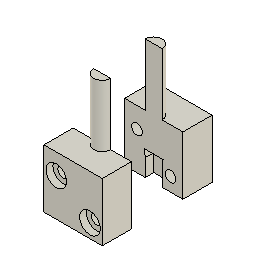
fl57sth76_gt2_adapter (Autodesk Fusion 360 design; units mm, degrees)
Autodesk Fusion 360 part; units mm, degrees
note: some values were not read from the file. Chosen so that the rebuilt part matches the saved one: which bodies a step acts on.
sketch "Sketch1" plane through (0, 0, 0) normal (0, 0, 1) x (1, 0, 0)
  line L0 (2.5, 2.5) -> (-2.5, 2.5)
  line L1 (-2.5, 2.5) -> (-2.5, -2.5)
  line L2 (-2.5, -2.5) -> (2.5, -2.5)
  line L3 (2.5, -2.5) -> (2.5, 2.5)
  line L4 (2.5, 2.5) -> (-2.5, -2.5) construction
  line L5 (-2.5, 2.5) -> (2.5, -2.5) construction
  dimension "d1" = 5
  dimension "d2" = 5
  constraint horizontal L0
  constraint perpendicular L0 L1
  constraint parallel L0 L2
  constraint parallel L1 L3
  constraint coincident L4 origin
  constraint coincident L5 origin
  measures "d1" distance of L1.end L2.end
  measures "d2" distance of L0.end L1.end
extrude "Extrude1" add sketch "Sketch1" along normal blind 5 makes body 1
ref_plane "WorkPlane1" through (0, 0, 7.15) normal (0, 0, 1) x (1, 0, 0)
sketch "Sketch2" plane through (0, 0, 7.15) normal (0, 0, 1) x (1, 0, 0)
  line L0 (2.675, 2.675) -> (-2.675, 2.675)
  line L1 (-2.675, 2.675) -> (-2.675, -2.675)
  line L2 (-2.675, -2.675) -> (2.675, -2.675)
  line L3 (2.675, -2.675) -> (2.675, 2.675)
  line L4 (2.675, 2.675) -> (-2.675, -2.675) construction
  line L5 (-2.675, 2.675) -> (2.675, -2.675) construction
  dimension "d7" = 5.35
  dimension "d8" = 5.35
  constraint horizontal L0
  constraint perpendicular L0 L1
  constraint parallel L0 L2
  constraint parallel L1 L3
  constraint coincident L4 origin
  constraint coincident L5 origin
  measures "d7" distance of L1.end L2.end
  measures "d8" distance of L0.end L1.end
loft "Loft1" add profiles "Sketch2" section 1 face at (-0.8333, 0.8333, 5) section 2 on bodies 1 bodies 1
sketch "Sketch3" plane through (0, 0, 0) normal (0, 0, 1) x (1, 0, 0)
  line L0 (8.5, 8.5) -> (-8.5, 8.5)
  line L1 (-8.5, 8.5) -> (-8.5, -8.5)
  line L2 (-8.5, -8.5) -> (8.5, -8.5)
  line L3 (8.5, -8.5) -> (8.5, 8.5)
  line L4 (8.5, 8.5) -> (-8.5, -8.5) construction
  line L5 (-8.5, 8.5) -> (8.5, -8.5) construction
  dimension "d9" = 17
  dimension "d10" = 17
  constraint horizontal L0
  constraint perpendicular L0 L1
  constraint parallel L0 L2
  constraint parallel L1 L3
  constraint coincident L4 origin
  constraint coincident L5 origin
  measures "d9" distance of L1.end L2.end
  measures "d10" distance of L0.end L1.end
extrude "Extrude2" add sketch "Sketch3" along normal blind 17 separate body makes body 2
combine "Combine1" operation cut target body 2 tool bodies 1
ref_plane "WorkPlane2" through (0, 0, 10) normal (0, 0, 1) x (1, 0, 0)
sketch "Sketch4" plane through (0, 0, 10) normal (0, 0, 1) x (1, 0, 0)
  line L0 (-4, -4) -> (4, -4)
  line L1 (4, -4) -> (4, 4)
  line L2 (4, 4) -> (-4, 4)
  line L3 (-4, 4) -> (-4, -4)
  line L4 (-4, -4) -> (4, 4) construction
  line L5 (4, -4) -> (-4, 4) construction
  dimension "d15" = 8
  dimension "d16" = 8
  constraint horizontal L0
  constraint perpendicular L0 L1
  constraint parallel L0 L2
  constraint parallel L1 L3
  constraint coincident L4 origin
  constraint coincident L5 origin
  measures "d15" distance of L1.end L2.end
  measures "d16" distance of L0.end L1.end
ref_plane "WorkPlane3" through (0, 0, 15) normal (0, 0, 1) x (1, 0, 0)
sketch "Sketch5" plane through (0, 0, 15) normal (0, 0, 1) x (1, 0, 0)
  line L0 (-3, 3) -> (3, 3)
  line L1 (3, 3) -> (3, -3)
  line L2 (3, -3) -> (-3, -3)
  line L3 (-3, -3) -> (-3, 3)
  line L4 (-3, 3) -> (3, -3) construction
  line L5 (3, 3) -> (-3, -3) construction
  dimension "d19" = 6
  dimension "d20" = 6
  constraint horizontal L0
  constraint perpendicular L0 L1
  constraint parallel L0 L2
  constraint parallel L1 L3
  constraint coincident L4 origin
  constraint coincident L5 origin
  measures "d19" distance of L1.end L2.end
  measures "d20" distance of L0.end L1.end
sketch "Sketch6" plane through (0, 0, 17) normal (0, 0, 1) x (-1, 0, 0)
  line L0 (-8.5, 8.5) -> (-8.5, -8.5)
  line L1 (-8.5, -8.5) -> (8.5, -8.5)
  line L2 (8.5, -8.5) -> (8.5, 8.5)
  line L3 (8.5, 8.5) -> (-8.5, 8.5)
  circle A0 centre (0, 0) radius 2.45
  dimension "d21" = 4.9
  constraint coincident A0.centre origin
  measures "d21" diameter of A0
extrude "Extrude3" add sketch "Sketch6" along normal blind 18 contours A0 bodies 2
hole "Hole1" at (4.9, -8.5, 4) direction (0, 1, 0) diameter 3.1 depth 43 tip angle 180 counterbore diameter 6 counterbore depth 2 bodies 2
hole "Hole2" at (-4.9, -8.5, 11) direction (0, 1, 0) diameter 3.1 depth 40 tip angle 180 counterbore diameter 6 counterbore depth 2 bodies 2
sketch "Sketch7" plane through (0, 8.5, 0) normal (0, 1, 0) x (-1, 0, 0)
  circle A0 centre (4.9, 11) radius 1.55
  circle A1 centre (-4.9, 4) radius 1.55
  line L0 (-8.5, 0) -> (8.5, 0)
  line L1 (8.5, 0) -> (8.5, 17)
  line L2 (8.5, 17) -> (-8.5, 17)
  line L3 (-8.5, 17) -> (-8.5, 0)
  line L4 (-3.3439, 1.1659) -> (-1.6676, 3.9306)
  line L5 (-1.6676, 3.9306) -> (-3.2237, 6.7646)
  line L6 (-3.2237, 6.7646) -> (-6.4561, 6.8341)
  line L7 (-6.4561, 6.8341) -> (-8.1324, 4.0694)
  line L8 (-8.1324, 4.0694) -> (-6.5763, 1.2354)
  line L9 (-6.5763, 1.2354) -> (-3.3439, 1.1659)
  line L10 (3.2834, 13.8) -> (1.6668, 11)
  line L11 (1.6668, 11) -> (3.2834, 8.2)
  line L12 (3.2834, 8.2) -> (6.5166, 8.2)
  line L13 (6.5166, 8.2) -> (8.1332, 11)
  line L14 (8.1332, 11) -> (6.5166, 13.8)
  line L15 (6.5166, 13.8) -> (3.2834, 13.8)
  point P0 (-4.9, 4)
  point P1 (4.9, 11)
  dimension "d38" = 2.8
  dimension "d39" = 2.8
  constraint coincident P0 A1.centre
  constraint coincident A0.centre P1
  measures "d38" distance of P0 L9
  measures "d39" distance of P1 L15
extrude "Extrude4" cut sketch "Sketch7" against normal blind 2.6 contours L4 L5 L6 L7 L8 L9 | L10 L11 L12 L13 L14 L15 bodies 2
ref_plane "WorkPlane4" through (0, 0, 8.5) normal (0, -1, 0) x (1, 0, 0)
split "Split1" by plane through (0, 0, 8.5) normal (0, -1, 0) bodies 2 makes body 3 at (3.6592, -8.5, 11.878)
move_body "Move1" bodies 3 to x (1, 0, 0) y (0, 1, 0) z (0, 0, 1) at (0, -10, 0)
move_body "Move2" bodies 3 to x (1, 0, 0) y (0, 1, 0) z (0, 0, 1) at (0, -5, 0)
equation "d38 = ( 5.6 / 2 ) * 1 mm"
equation "d42 = ( -17 / 2 ) * 1 mm"
